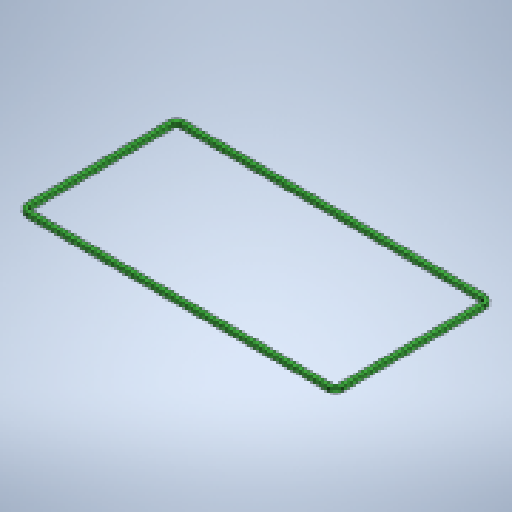
# Autodesk Inventor part: PinecilCaseBorder
Saved by Autodesk Inventor 2026 (Build 300175050, 175E)
## iProperties
Created: 2025-10-10
Part Number: PinecilCaseBorder
Material: ABS Plastic
Document SubType Name: Modeling
Designer: Nicholas M
Density: 1.06 g/cm^3
Appearance: Smooth - Dark Forest Green
Author: Nicholas M
Autodesk Inventor part; units mm, degrees
ref_plane "YZ Plane" through (0, 0, 0) normal (1, 0, 0) x (0, 1, 0)
ref_plane "XZ Plane" through (0, 0, 0) normal (0, 1, 0) x (-1, 0, 0)
ref_plane "XY Plane" through (0, 0, 0) normal (0, 0, 1) x (1, 0, 0)
sketch "Sketch1" plane through (0, 0, 0) normal (0, 1, 0) x (-1, 0, 0)
  line L0 (3.175, 0) -> (123.825, 0)
  line L1 (127, -3.175) -> (127, -60.325)
  line L2 (123.825, -63.5) -> (3.175, -63.5)
  line L3 (0, -60.325) -> (0, -3.175)
  arc A0 (127, -3.175) -> (123.825, 0) centre (123.825, -3.175) ccw
  arc A1 (123.825, -63.5) -> (127, -60.325) centre (123.825, -60.325) ccw
  arc A2 (0, -60.325) -> (3.175, -63.5) centre (3.175, -60.325) ccw
  arc A3 (3.175, 0) -> (0, -3.175) centre (3.175, -3.175) ccw
  line L4 (1.905, -3.175) -> (1.905, -60.325)
  arc A4 (1.905, -60.325) -> (3.175, -61.595) centre (3.175, -60.325) ccw
  line L5 (3.175, -61.595) -> (123.825, -61.595)
  arc A5 (123.825, -61.595) -> (125.095, -60.325) centre (123.825, -60.325) ccw
  line L6 (125.095, -60.325) -> (125.095, -3.175)
  arc A6 (125.095, -3.175) -> (123.825, -1.905) centre (123.825, -3.175) ccw
  line L7 (123.825, -1.905) -> (3.175, -1.905)
  arc A7 (3.175, -1.905) -> (1.905, -3.175) centre (3.175, -3.175) ccw
  point P0 (0, 0)
  point P1 (127, -63.5)
  point P2 (127, 0)
  point P3 (0, -63.5)
  point P4 (3.175, -3.175)
  point P5 (123.825, -3.175)
  point P6 (123.825, -60.325)
  point P7 (3.175, -60.325)
  dimension "d0" = 63.5
  dimension "d1" = 127
  dimension "d2" = 3.175
  dimension "d3" = 3.175
  dimension "d7" = 1.905
  constraints: 16 end point, 16 point on circle, 8 centre point, 8 point on line, 8 tangent, 4 parallel, 2 equal radius, 2 perpendicular, 1 horizontal, 7 other
  measures "d0" distance of point (127, 0) point (127, -63.5)
  measures "d1" distance of point (127, -63.5) point (0, -63.5)
  measures "d2" radius of A0
  measures "d3" radius of A3
  measures "d7" radial gap between concentric circles of A3 A7
extrude "Extrusion1" add sketch "Sketch1" along normal blind 1.5875
equation "\"d3\" = d2"
body "Solid1"
